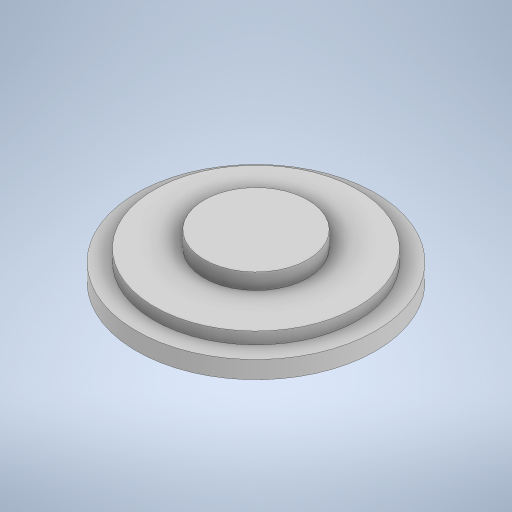
# Autodesk Inventor part: 스피커
Saved by Autodesk Inventor 2023 (Build 270158000, 158)
## iProperties
Created: 2022-11-10
Part Number: 스피커
Material: 일반
Document SubType Name: Modeling
Designer: user
Density: 1 g/cm^3
Appearance: 기본값
Author: user
Autodesk Inventor part; units mm, degrees
ref_plane "YZ Plane" through (0, 0, 0) normal (1, 0, 0) x (0, 1, 0)
ref_plane "XZ Plane" through (0, 0, 0) normal (0, 1, 0) x (-1, 0, 0)
ref_plane "XY Plane" through (0, 0, 0) normal (0, 0, 1) x (1, 0, 0)
sketch "스케치1" plane through (0, 0, 0) normal (0, 0, 1) x (1, 0, 0)
  line L0 (0, 0) -> (15, 0)
  line L1 (15, 0) -> (15, 2.2)
  line L2 (15, 2.2) -> (12.75, 2.2)
  line L3 (12.75, 2.2) -> (12.75, 3.7)
  line L4 (12.75, 3.7) -> (6.5, 3.7)
  line L5 (6.5, 3.7) -> (6.5, 5.7)
  line L6 (6.5, 5.7) -> (0, 5.7)
  line L7 (0, 8.3) -> (0, 0)
  dimension "d0" = 30
  dimension "d1" = 25.5
  dimension "d2" = 13
  dimension "d4" = 2.2
  dimension "d5" = 1.5
  dimension "d6" = 2
  constraints: 16 end point, 6 perpendicular, 1 horizontal, 1 point on line
  measures "d0" diameter of L1 L7
  measures "d1" diameter of L3.end L7
  measures "d2" diameter of L5 L7
  measures "d4" distance between parallel lines of L0 L2
  measures "d5" distance of L2.end L3.end
  measures "d6" distance of L4.end L5.end
revolve "회전1" add sketch "스케치1" angle 360 about axis through (0, 8.3, 0) along (0, -1, 0)
